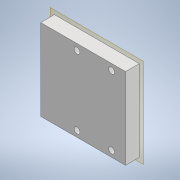
# Autodesk Inventor part: spacer_plate
Saved by Autodesk Inventor 2022 (Build 260153000, 153)
## iProperties
Created: 2021-07-14
Part Number: spacer_plate
Material: Generic
Document SubType Name: Modeling
Designer: gfellows
Density: 1 g/cm^3
Appearance: Default
Author: gfellows
Autodesk Inventor part; units mm, degrees
ref_plane "YZ Plane" through (0, 0, 0) normal (1, 0, 0) x (0, 1, 0)
ref_plane "XZ Plane" through (0, 0, 0) normal (0, 1, 0) x (-1, 0, 0)
ref_plane "XY Plane" through (0, 0, 0) normal (0, 0, 1) x (1, 0, 0)
ref_plane "Work Plane1" through (175.2465, 19.25, 68.825) normal (0, 0, 1) x (0, 1, 0)
sketch "Sketch1" plane through (175.2465, 19.25, 68.825) normal (0, 0, 1) x (0, 1, 0)
  line L0 (-37.846, -0.254) -> (-0.254, -0.254) projected
  line L1 (-37.846, -39.497) -> (-37.846, -0.254) projected
  line L2 (-0.254, -39.497) -> (-37.846, -39.497) projected
  line L3 (-0.254, -0.254) -> (-0.254, -39.497) projected
  circle A0 centre (-35.05, -33.02) radius 1.3525 projected
  circle A1 centre (-35.05, -17.02) radius 1.3525 projected
  circle A2 centre (-3.05, -33.02) radius 1.3525 projected
  circle A3 centre (-3.05, -17.02) radius 1.3525 projected
  point P0 (-19.25, 175.2465)
extrude "Extrusion1" add sketch "Sketch1" along normal blind 6.35
body "Solid1"
